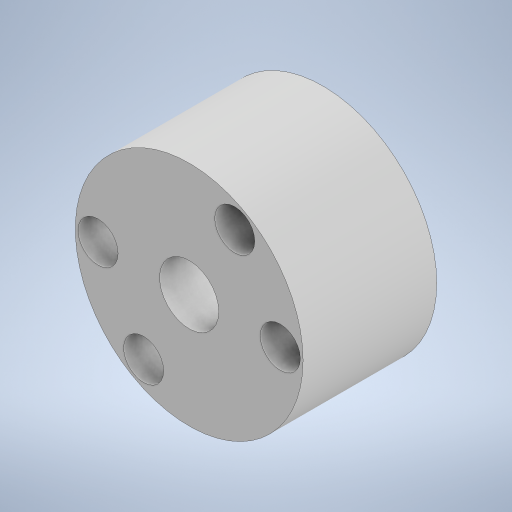
# Autodesk Inventor part: Crankshaft
Saved by Autodesk Inventor 2023 (Build 270158000, 158)
## iProperties
Created: 2022-10-29
Part Number: Crankshaft
Material: Generic
Document SubType Name: Modeling
Designer: tommy
Density: 1 g/cm^3
Appearance: Default
Author: tommy
Autodesk Inventor part; units mm, degrees
ref_plane "YZ Plane" through (0, 0, 0) normal (1, 0, 0) x (0, 1, 0)
ref_plane "XZ Plane" through (0, 0, 0) normal (0, 1, 0) x (-1, 0, 0)
ref_plane "XY Plane" through (0, 0, 0) normal (0, 0, 1) x (1, 0, 0)
sketch "Sketch1" plane through (0, 0, 0) normal (0, 0, 1) x (1, 0, 0)
  circle A0 centre (7.62, 0) radius 1.6764
  circle A1 centre (-7.62, 0) radius 1.6764
  circle A2 centre (0, 0) radius 9.525
  circle A3 centre (-3.81, -6.5991) radius 1.6764
  circle A4 centre (3.81, 6.5991) radius 1.6764
  circle A5 centre (0, 0) radius 2.4765
  point P0 (-4.7625, -8.2489)
  point P1 (4.7625, 8.2489)
  dimension "d69" = 3.3528
  dimension "d70" = 3.3528
  dimension "d75" = 3.3528
  dimension "d76" = 3.3528
  dimension "d79" = 7.62
  dimension "d80" = 7.62
  dimension "d82" = 4.953
  dimension "d83" = 7.62
  dimension "d84" = 7.62
  constraints: 5 centre point, 5 coincident, 3 other
  measures "d69" diameter of A1
  measures "d70" diameter of A0
  measures "d75" diameter of A4
  measures "d76" diameter of A3
  measures "d79" distance of A4.centre point (0, 0)
  measures "d80" distance of point (0, 0) A3.centre
  measures "d82" diameter of A5
  measures "d83" distance of point (0, 0) A0.centre
  measures "d84" distance of point (0, 0) A1.centre
extrude "Extrusion14" add sketch "Sketch1" along normal blind 11.176
body "Solid5"
